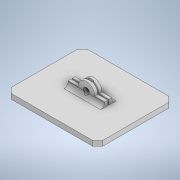
# Autodesk Inventor part: 테스트용 고정판
Saved by Autodesk Inventor 2022.2 (Build 262287010, 287A)
## iProperties
Created: 2022-04-11
Part Number: 테스트용 고정판
Material: 일반
Document SubType Name: Modeling
Designer: USER
Density: 1 g/cm^3
Appearance: 기본값
Author: USER
Autodesk Inventor part; units mm, degrees
ref_plane "YZ Plane" through (0, 0, 0) normal (1, 0, 0) x (0, 1, 0)
ref_plane "XZ Plane" through (0, 0, 0) normal (0, 1, 0) x (-1, 0, 0)
ref_plane "XY Plane" through (0, 0, 0) normal (0, 0, 1) x (1, 0, 0)
sketch "스케치1" plane through (0, 0, 0) normal (0, 0, 1) x (1, 0, 0)
  circle A0 centre (0, 0) radius 5.4
  line L0 (-35.9747, -10.4) -> (35.9747, -10.4)
  circle A1 centre (0, 0) radius 13 construction
  arc A2 (15.9747, -0.9) -> (-15.9747, -0.9) centre (0, 0) ccw
  line L1 (-16, -10.4) -> (-26.4, -10.4)
  line L2 (0, 0) -> (0, -3.1223) construction
  line L3 (-35.9747, -0.9) -> (-15.9747, -0.9)
  line L4 (-35.9747, -0.9) -> (-35.9747, -10.4)
  line L5 (35.9747, -0.9) -> (15.9747, -0.9)
  line L6 (35.9747, -0.9) -> (35.9747, -10.4)
  point P0 (0, -13.3333)
  point P1 (0, -5.4)
  point P2 (26.4, -10.4)
  point P3 (0, -10.4)
  point P4 (-15.9905, 0.5521)
  point P5 (15.9905, 0.5521)
  dimension "d0" = 10.8
  dimension "d51" = 5
  dimension "d73" = 3
  dimension "d74" = 26
  dimension "d83" = 9.5
  dimension "d84" = 20
  constraints: 14 end point, 5 point on circle, 5 symmetric about line, 4 coincident, 4 vertical alignment, 3 point on line, 2 centre point, 2 horizontal, 2 vertical, 1 midpoint, 2 other
  measures "d51" distance from line of point (0, -5.4) L0
  measures "d73" radial gap between concentric circles of A1 A2
  measures "d74" diameter of A1
  measures "d83" distance between parallel lines of L3 L0
  measures "d84" distance of L3.start L3.end
extrude "돌출1" add sketch "스케치1" along normal mid plane 14
chamfer "모따기6" distance 0.3 angle 45 2 edges at (-5.4, 0, 7) (-5.4, 0, -7)
sketch "스케치7" plane through (-26.4, -10.4, 7) normal (0, -1, 0) x (1, 0, 0)
  line L0 (-63.6, 68) -> (116.4, 68)
  line L1 (116.4, 68) -> (116.4, -82)
  line L2 (116.4, -82) -> (-63.6, -82)
  line L3 (-63.6, -82) -> (-63.6, 68)
  line L4 (-63.6, 68) -> (116.4, -82) construction
  line L5 (116.4, 68) -> (-63.6, -82) construction
  point P0 (26.4, -7)
  dimension "d54" = 180
  dimension "d55" = 150
  constraints: 12 end point, 2 midpoint, 2 parallel, 1 horizontal, 1 perpendicular
  measures "d54" distance of L1.end L2.end
  measures "d55" distance of L0.end L1.end
extrude "돌출7" add sketch "스케치7" along normal blind 10
fillet "모깎기7" radius 8 2 edges at (0, -10.4, 7) (0, -10.4, -7)
chamfer "모따기8" distance 10 angle 45 4 edges at (90, -15.4, -75) (90, -15.4, 75) (-90, -15.4, 75) (-90, -15.4, -75)
ref_plane "작업 평면1" through (0, 16, 0) normal (0, 1, 0) x (1, 0, 0)
sketch "스케치10" plane through (0, 16, 0) normal (0, 1, 0) x (1, 0, 0)
  line L0 (-5.35, 2.15) -> (5.35, 2.15)
  line L1 (5.35, 2.15) -> (5.35, -2.15)
  line L2 (5.35, -2.15) -> (-5.35, -2.15)
  line L3 (-5.35, -2.15) -> (-5.35, 2.15)
  line L4 (-5.35, 2.15) -> (5.35, -2.15) construction
  line L5 (5.35, 2.15) -> (-5.35, -2.15) construction
  point P0 (0, 0)
  dimension "d76" = 10.7
  dimension "d77" = 4.3
  constraints: 12 end point, 2 midpoint, 2 parallel, 1 horizontal, 1 perpendicular
  measures "d76" distance of L1.end L2.end
  measures "d77" distance of L0.end L1.end
extrude "돌출10" cut sketch "스케치10" against normal blind 16
sketch "스케치11" plane through (0, 0, 0) normal (1, 0, 0) x (0, 1, 0)
  line L0 (-10.4, -65) -> (-10.4, 65) projected
  line L1 (-10.4, -1.15) -> (18.3828, -1.15)
  line L2 (18.3828, -1.15) -> (18.3828, 1.15)
  line L3 (18.3828, 1.15) -> (-10.4, 1.15)
  line L4 (-10.4, 1.15) -> (-10.4, -1.15)
  point P0 (0, 0)
  point P1 (18.3828, 0)
  dimension "d80" = 2.3
  constraints: 8 end point, 2 parallel, 1 horizontal, 1 horizontal alignment, 1 midpoint, 1 perpendicular, 1 point on line
  measures "d80" distance of L1.end L2.end
extrude "돌출11" cut sketch "스케치11" along normal through all both and the other way through all
